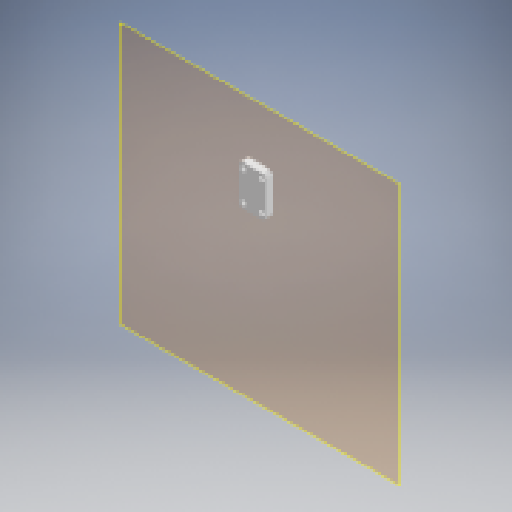
# Autodesk Inventor part: Подставка под солноид
Saved by Autodesk Inventor 2023 (Build 270158000, 158)
## iProperties
Created: 2025-04-10
Part Number: Подставка под солноид
Material: Типовые
Document SubType Name: Modeling
Designer: Ivan
Density: 1 g/cm^3
Appearance: По умолчанию
Author: Ivan
Autodesk Inventor part; units mm, degrees
ref_plane "YZ Plane" through (0, 0, 0) normal (1, 0, 0) x (0, 1, 0)
ref_plane "XZ Plane" through (0, 0, 0) normal (0, 1, 0) x (-1, 0, 0)
ref_plane "XY Plane" through (0, 0, 0) normal (0, 0, 1) x (1, 0, 0)
ref_plane "РабПлоскость1" through (0, 0, 0) normal (0, 0, 1) x (1, 0, 0)
sketch "Эскиз1" plane through (0, 0, 0) normal (0, 0, 1) x (1, 0, 0)
  circle A0 centre (7.416, 59.491) radius 2 projected
  circle A1 centre (7.416, 35.509) radius 2 projected
  circle A2 centre (-7.416, 35.509) radius 2 projected
  circle A3 centre (-7.416, 59.491) radius 2 projected
  line L0 (11, 64.0958) -> (-11, 64.0958)
  line L1 (-11, 64.0958) -> (-11, 30.9042)
  line L2 (-11, 30.9042) -> (11, 30.9042)
  line L3 (11, 30.9042) -> (11, 64.0958)
  line L4 (11, 64.0958) -> (-11, 30.9042) construction
  line L5 (7.416, 59.491) -> (-7.416, 35.509) construction
  arc A4 (-24.6917, 37.0776) -> (24.6917, 37.0776) centre (0, 73.5704) ccw projected
  point P0 (0, 0)
  point P1 (0, 47.5)
  dimension "d0" = 22
  constraints: 12 end point, 2 midpoint, 2 parallel, 1 horizontal, 1 perpendicular, 1 point on circle
  measures "d0" distance of L2.end L1.end
extrude "Выдавливание1" add sketch "Эскиз1" along normal blind 6 contours L3 L2 L1 L0
fillet "Сопряжение1" radius 3.5 4 edges at (-11, 30.9042, 3) (11, 30.9042, 3) (11, 64.0958, 3) (-11, 64.0958, 3)
